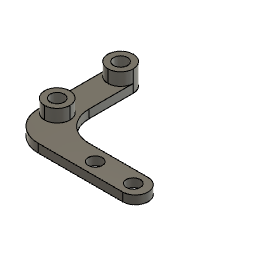
upper sensor holder v1 (Autodesk Fusion 360 design; units mm, degrees)
Autodesk Fusion 360 part; units mm, degrees
note: some values were not read from the file. Set by a fixed rule: which sketch regions a step uses.
sketch "Sketch1" plane through (0, 0, 0) normal (0, 1, 0) x (1, 0, 0)
  circle A0 centre (-4.5, 0) radius 1.65
  circle A1 centre (4.5, 0) radius 1.65
  line L0 (-8, -3) -> (8, -3)
  line L1 (8, -3) -> (8, 3)
  line L2 (8, 3) -> (-8, 3)
  circle A2 centre (-19, 5.5) radius 1.65
  circle A3 centre (-19, 20.5) radius 1.65
  line L3 (-22, 23.5) -> (-16, 23.5)
  line L4 (-16, 23.5) -> (-16, 2.5)
  line L5 (-16, 2.5) -> (-22, 2.5)
  line L6 (-22, 2.5) -> (-22, 23.5)
  line L7 (-8, -3) -> (-22, -3)
  line L8 (-22, -3) -> (-22, 3)
  line L9 (-22, 3) -> (-8, 3)
  line L10 (-22, 23.5) -> (-16, 23.5)
  line L11 (-16, 23.5) -> (-16, 17.5)
  line L12 (-16, 17.5) -> (-22, 17.5)
  line L13 (-22, 17.5) -> (-22, 23.5)
  line L14 (-16, 2.5) -> (-22, 2.5)
  line L15 (-22, 2.5) -> (-22, 8.5)
  line L16 (-22, 8.5) -> (-16, 8.5)
  line L17 (-16, 8.5) -> (-16, 2.5)
  dimension "d1" = 3.3
  dimension "d2" = 3.3
  dimension "d3" = 4.5
  dimension "d4" = 4.5
  dimension "d5" = 3.3
  dimension "d6" = 3.3
  dimension "d7" = 19
  dimension "d8" = 15
  dimension "d9" = 5.5
  dimension "d10" = 6
  dimension "d16" = 3
  dimension "d17" = 3
  dimension "d18" = 3
  dimension "d19" = 3
  dimension "d20" = 3
  dimension "d21" = 3
  constraint horizontal L0
  constraint vertical L1
  constraint horizontal L2
  constraint vertical A2.centre A3.centre
  constraint horizontal L3
  constraint vertical L4
  constraint horizontal L5
  constraint vertical L6
  constraint horizontal L7
  constraint vertical L8
  constraint horizontal L9
  constraint coincident L6 L8.end
  constraint horizontal L10
  constraint vertical L11
  constraint horizontal L12
  constraint vertical L13
  constraint coincident L4 L11.end
  constraint horizontal L14
  constraint vertical L15
  constraint horizontal L16
  constraint vertical L17
  constraint coincident L6 L15.end
  measures "d1" diameter of A0
  measures "d2" diameter of A1
  measures "d3" distance of origin A1.centre
  measures "d4" distance of origin A0.centre
  measures "d5" diameter of A2
  measures "d6" diameter of A3
  measures "d7" horizontal distance of origin A2.centre
  measures "d8" distance of A2.centre A3.centre
  measures "d9" distance of origin A2.centre A0.centre
  measures "d10" distance of L0 L2
  measures "d16" distance of A2.centre L5
  measures "d17" distance of A2.centre L16
  measures "d18" distance of A3.centre L12
  measures "d19" distance of A3.centre L10
  measures "d20" distance of A3.centre L4
  measures "d21" distance of A3.centre L6
extrude "Extrude2" add sketch "Sketch1" along normal blind 5 contours L4 L5 L6 L8 L9 L14 L15 L17 | L4 L6 L9 L15 L16 L17 | L3 L4 L6 L10 L11 L12 L13 makes body 1 at (-17.3521, 3.3333, -5.4178) makes body 2 at (-17.3521, 3.3333, -20.4178)
extrude "Extrude1" add sketch "Sketch1" along normal blind 2 contours L0 L1 L2 L4 L5 L7 L8 L9 L14 L17 | L4 L5 L6 L8 L9 L14 L15 L17 | L4 L6 L12 L16 bodies 1 2
fillet "Fillet1" radius 3 10 edges at (-22, 3.5, -2.5) (-22, 3.5, -8.5) (-22, 3.5, -17.5) (-22, 2.5, -23.5) (-16, 3.5, -17.5) (-16, 3.5, -2.5) (8, 1, 3) (8, 1, -3) (-16, 3.5, -8.5) (-16, 2.5, -23.5) on bodies 1
fillet "Fillet2" radius 7 1 edges at (-17.3417, 1, -3) on bodies 1
fillet "Fillet3" radius 7 1 edges at (-22, 1, 3) on bodies 1
equation "d4 = d3"
